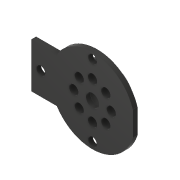
# Autodesk Inventor part: Small Heater Holder for Use With Fan
Saved by Autodesk Inventor 2017 (Build 210142000, 142)
## iProperties
Created: 2016-09-26
Part Number: Small Heater Holder for Use With Fan
Material: Generic
Document SubType Name: Modeling
Designer: ge937963
Density: 1 g/cm^3
Appearance: Smooth - Black
Author: ge937963
Autodesk Inventor part; units mm, degrees
ref_plane "YZ Plane" through (0, 0, 0) normal (1, 0, 0) x (0, 1, 0)
ref_plane "XZ Plane" through (0, 0, 0) normal (0, 1, 0) x (-1, 0, 0)
ref_plane "XY Plane" through (0, 0, 0) normal (0, 0, 1) x (1, 0, 0)
sketch "Sketch1" plane through (0, 0, 0) normal (0, 0, 1) x (1, 0, 0)
  circle A0 centre (4.5902, 12.1566) radius 1.27 projected
  circle A1 centre (4.5902, -12.1619) radius 1.27 projected
  circle A2 centre (-12.9763, 0.0036) radius 1.27 projected
  line L0 (18.2524, -4.1824) -> (18.2524, 4.1791) projected
  arc A3 (18.2524, 4.1791) -> (-7.4923, 7.6236) centre (4.5902, -0.0017) ccw projected
  line L1 (-7.4923, 7.6236) -> (-16.1513, 7.6236) projected
  line L2 (-16.1513, 7.6236) -> (-16.1513, -7.6164) projected
  line L3 (-16.1513, -7.6164) -> (-7.4989, -7.6164) projected
  arc A4 (-7.4989, -7.6164) -> (18.2524, -4.1824) centre (4.5902, -0.0017) ccw projected
  line L4 (-4.9271, -3.1767) -> (-8.2305, -3.1767) projected
  arc A5 (-8.2305, 3.1733) -> (-8.2305, -3.1767) centre (4.5902, -0.0017) ccw projected
  line L5 (-8.2305, 3.1733) -> (-4.9271, 3.1733) projected
  arc A6 (-4.9271, -3.1767) -> (-4.9271, 3.1733) centre (4.5902, -0.0017) ccw projected
  circle A7 centre (4.5902, -0.0017) radius 3.175 projected
  circle A8 centre (4.5902, -0.0017) radius 9.017
  circle A9 centre (4.5902, -0.0017) radius 4.953
  point P0 (0, 0)
  dimension "d0" = 1.778
  dimension "d1" = 1.016
  constraints: 2 centre point, 2 coincident
  measures "d0" radial gap between concentric circles of A7 A9
  measures "d1" radial gap between concentric circles of A8 A6
extrude "Extrusion1" add sketch "Sketch1" against normal blind 19.05 contours A8
sketch "Sketch2" plane through (4.5902, -0.0017, 0) normal (0, 0, 1) x (1, 0, 0)
  circle A0 centre (0, 0) radius 4.953 projected
  point P0 (-4.5902, 0.0017)
extrude "Extrusion2" add sketch "Sketch2" against normal blind 7.62
sketch "Sketch3" plane through (0, 0, 0) normal (1, 0, 0) x (0, 1, 0)
  line L0 (3.1733, -8.4292) -> (-3.1767, -8.4292) projected
  point P0 (0, 0)
sketch "Sketch5" plane through (4.5902, -0.0017, 0) normal (0, 0, 1) x (1, 0, 0)
  circle A0 centre (0, 12.1583) radius 1.27 projected
  circle A1 centre (0, -12.1603) radius 1.27 projected
  circle A2 centre (-17.5665, 0.0053) radius 1.27 projected
  line L0 (13.6621, -4.1808) -> (13.6621, 4.1808) projected
  arc A3 (13.6621, 4.1808) -> (-12.0826, 7.6253) centre (0, 0) ccw projected
  line L1 (-12.0826, 7.6253) -> (-20.7415, 7.6253) projected
  line L2 (-20.7415, 7.6253) -> (-20.7415, -7.6147) projected
  line L3 (-20.7415, -7.6147) -> (-12.0892, -7.6147) projected
  arc A4 (-12.0892, -7.6147) -> (13.6621, -4.1808) centre (0, 0) ccw projected
  line L4 (-9.5174, -3.175) -> (-12.8207, -3.175) projected
  arc A5 (-12.8207, 3.175) -> (-12.8207, -3.175) centre (0, 0) ccw projected
  line L5 (-12.8207, 3.175) -> (-9.5174, 3.175) projected
  arc A6 (-9.5174, -3.175) -> (-9.5174, 3.175) centre (0, 0) ccw projected
  point P0 (-4.5902, 0.0017)
extrude "Extrusion4" add sketch "Sketch5" along normal blind 1.5875 contours A4 L3 L2 L1 A3 L0 | L4 A5 L5 A6
sketch "Sketch6" plane through (4.5902, -0.0017, 1.5875) normal (0, 0, 1) x (1, 0, 0)
  circle A0 centre (0, -12.1603) radius 1.27 projected
  circle A1 centre (0, -12.1603) radius 1.524
  circle A2 centre (-17.5665, 0.0053) radius 1.27 projected
  circle A3 centre (-17.5665, 0.0053) radius 1.524
  circle A4 centre (0, 12.1583) radius 1.27 projected
  circle A5 centre (0, 12.1583) radius 1.524
  point P0 (-4.5902, 0.0017)
  dimension "d12" = 3.048
  constraints: 3 centre point, 3 coincident, 2 equal radius
  measures "d12" diameter of A1
extrude "Extrusion5" cut sketch "Sketch6" against normal blind 1.5875
sketch "Sketch7" plane through (4.5902, -0.0017, -7.62) normal (0, 0, -1) x (-1, 0, 0)
  circle A0 centre (0, 0) radius 3.429
  point P0 (4.5902, 0.0017)
  dimension "d15" = 6.858
  constraints: 1 centre point
  measures "d15" diameter of A0
extrude "Extrusion6" cut sketch "Sketch7" against normal up to surface (7.62 mm away)
sketch "Sketch8" plane through (0, 0, 0) normal (0, 1, 0) x (-1, 0, 0)
  spline S0 degree 3 poles (-8.0192, -14.5252) (-8.0192, -14.0929) (-7.9325, -13.6329) (-7.5821, -12.7886) (-7.3185, -12.4041) (-6.7114, -11.797) (-6.3268, -11.5333) (-5.4824, -11.1829) (-5.0225, -11.0962) (-4.158, -11.0962) (-3.698, -11.1829) (-2.8537, -11.5333) (-2.4691, -11.797) (-1.862, -12.4041) (-1.5984, -12.7886) (-1.248, -13.6329) (-1.1612, -14.0929) (-1.1612, -14.9574) (-1.248, -15.4174) (-1.5984, -16.2617) (-1.862, -16.6463) (-2.4691, -17.2534) (-2.8537, -17.517) (-3.698, -17.8675) (-4.158, -17.9542) (-5.0225, -17.9542) (-5.4824, -17.8675) (-6.3268, -17.517) (-6.7114, -17.2534) (-7.3185, -16.6463) (-7.5821, -16.2617) (-7.9325, -15.4174) (-8.0192, -14.9574) (-8.0192, -14.5252) knots 0 0 0 0 0.129682 0.129682 0.259363 0.259363 0.389031 0.389031 0.5187 0.5187 0.648368 0.648368 0.778036 0.778036 0.907718 0.907718 1.037399 1.037399 1.167081 1.167081 1.296762 1.296762 1.426431 1.426431 1.556099 1.556099 1.685767 1.685767 1.815435 1.815435 1.945117 1.945117 2.074799 2.074799 2.074799 2.074799 projected
  point P0 (0, 0)
  point P1 (-8.0192, -14.5252)
extrude "Extrusion7" cut sketch "Sketch8" against normal blind 25.4
sketch "Sketch9" plane through (0, 0, 0) normal (1, 0, 0) x (0, 1, 0)
  line L0 (6.3536, -8.255) -> (-6.3464, -8.255) projected
  line L1 (-5.4574, -16.7982) -> (5.4646, -16.7982) projected
  line L2 (5.4646, -8.255) -> (5.4646, -66.0222) projected
  line L3 (-5.4574, -66.0222) -> (-5.4574, -8.255) projected
  line L4 (4.9513, -7.62) -> (4.9513, -19.05) projected
  line L5 (4.9513, -8.255) -> (-5.4574, -8.255)
  line L6 (-5.4574, -8.255) -> (-5.4574, -16.7982)
  line L7 (-5.4574, -16.7982) -> (4.9513, -16.7982)
  line L8 (4.9513, -16.7982) -> (4.9513, -8.255)
  line L9 (4.0885, -8.255) -> (-4.122, -8.255)
  line L10 (-4.122, -8.255) -> (-4.122, -14.2031)
  line L11 (-4.122, -14.2031) -> (4.0885, -14.2031)
  line L12 (4.0885, -14.2031) -> (4.0885, -8.255)
  line L13 (3.81, -8.255) -> (-3.81, -8.255)
  line L14 (-3.81, -8.255) -> (-3.81, -14.605)
  line L15 (-3.81, -14.605) -> (3.81, -14.605)
  line L16 (3.81, -14.605) -> (3.81, -8.255)
  point P0 (0, 0)
  point P1 (0, -14.605)
  dimension "d22" = 6.35
  dimension "d23" = 7.62
  constraints: 24 end point, 6 parallel, 4 point on line, 3 horizontal, 3 perpendicular, 1 midpoint, 1 vertical alignment
  measures "d22" distance of L13.end L14.end
  measures "d23" distance between parallel lines of L16 L14
extrude "Extrusion8" cut sketch "Sketch9" along normal mid plane 12.7 contours L16 L11 L14 L0 | L16 L15 L14 L11
sketch "Sketch10" plane through (4.5902, -0.0017, 1.5875) normal (0, 0, 1) x (1, 0, 0)
  circle A0 centre (0, 0) radius 3.429 projected
  circle A1 centre (0, 0) radius 2.2479
  point P0 (-4.5902, 0.0017)
  dimension "d24" = 4.4958
  constraints: 1 centre point, 1 coincident
  measures "d24" diameter of A1
extrude "Extrusion9" cut sketch "Sketch10" against normal blind 25.4 contours A1
sketch "Sketch11" plane through (4.5902, -0.0017, -7.62) normal (0, 0, -1) x (-1, 0, 0)
  circle A0 centre (0, 0) radius 4.953
  point P0 (4.5902, 0.0017)
  constraints: 1 centre point
extrude "Extrusion10" cut sketch "Sketch11" against normal blind 3.81
sketch "Sketch12" plane through (4.5902, -0.0017, -19.05) normal (0, 0, -1) x (-1, 0, 0)
  circle A0 centre (0, 0) radius 2.2479 projected
  circle A1 centre (0, 0) radius 36.9649
  point P0 (4.5902, 0.0017)
  constraints: 1 centre point, 1 coincident
extrude "Extrusion11" cut sketch "Sketch12" against normal up to surface (15.24 mm away)
sketch "Sketch13" plane through (4.5902, -0.0017, -3.81) normal (0, 0, -1) x (-1, 0, 0)
  circle A0 centre (6.3764, 0.0017) radius 1.5875
  point P0 (4.5902, 0.0017)
  dimension "d31" = 3.175
  constraints: 1 centre point
  measures "d31" diameter of A0
extrude "Extrusion12" cut sketch "Sketch13" against normal blind 25.4
pattern_circular "Circular Pattern1" count 8 over 360 about axis through (4.5902, -0.0017, 1.5875) along (0, 0, -1) of "Extrusion12"
body "Solid1"
